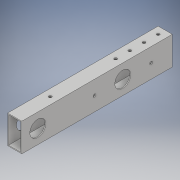
# Autodesk Inventor part: 1X2 7in
Saved by Autodesk Inventor 2018 (Build 220112000, 112)
## iProperties
Created: 2019-01-11
Material: Generic
Document SubType Name: Modeling
Designer: s-2512711
Density: 1 g/cm^3
Appearance: Default
Author: s-2512711
Autodesk Inventor part; units mm, degrees
ref_plane "YZ Plane" through (0, 0, 0) normal (1, 0, 0) x (0, 1, 0)
ref_plane "XZ Plane" through (0, 0, 0) normal (0, 1, 0) x (-1, 0, 0)
ref_plane "XY Plane" through (0, 0, 0) normal (0, 0, 1) x (1, 0, 0)
sketch "Sketch1" plane through (0, 0, 0) normal (0, 0, 1) x (1, 0, 0)
  line L0 (0, 0) -> (25.4, 0)
  line L1 (25.4, 0) -> (25.4, 50.8)
  line L2 (25.4, 50.8) -> (0, 50.8)
  line L3 (0, 50.8) -> (0, 0)
  line L4 (1.5875, 49.2125) -> (23.8125, 49.2125)
  line L5 (23.8125, 49.2125) -> (23.8125, 1.5875)
  line L6 (23.8125, 1.5875) -> (1.5875, 1.5875)
  line L7 (1.5875, 1.5875) -> (1.5875, 49.2125)
  dimension "d0" = 25.4
  dimension "d1" = 50.8
  dimension "d2" = 1.5875
  constraints: 16 end point, 4 parallel, 2 perpendicular, 1 horizontal, 3 other
  measures "d0" distance of L2.end L1.end
  measures "d1" distance of L1.end L0.end
  measures "d2" distance between parallel lines of L2 L4
extrude "Extrusion1" add sketch "Sketch1" along normal blind 269.875
sketch "Sketch2" plane through (25.4, 0, 0) normal (1, 0, 0) x (0, 0, -1)
  line L0 (-269.875, 49.2125) -> (-269.875, 1.5875) construction
  line L1 (-269.875, 25.4) -> (-241.3, 25.4) construction
  circle A0 centre (-241.3, 25.4) radius 14.2875
  point P0 (0, 0)
  dimension "d20" = 28.575
  dimension "d21" = 28.575
  constraints: 2 end point, 1 centre point, 1 coincident, 1 horizontal, 1 midpoint
  measures "d20" distance of L1.start L1.end
  measures "d21" diameter of A0
sketch "Sketch4" plane through (0, 50.8, 0) normal (0, 1, 0) x (1, 0, 0)
  line L0 (1.5875, 0) -> (23.8125, 0) construction
  line L1 (12.7, 0) -> (12.7, -12.7) construction
  line L2 (12.7, -12.7) -> (12.7, -38.1) construction
  line L3 (12.7, -38.1) -> (12.7, -63.5) construction
  circle A0 centre (12.7, -12.7) radius 2.5797
  circle A1 centre (12.7, -38.1) radius 2.5797
  circle A2 centre (12.7, -63.5) radius 2.5797
  point P0 (0, 0)
  dimension "d14" = 12.7
  dimension "d15" = 25.4
  dimension "d16" = 25.4
  dimension "d17" = 5.1594
  constraints: 6 end point, 3 centre point, 3 coincident, 2 point on line, 1 midpoint, 1 vertical
  measures "d14" distance of L1.start L1.end
  measures "d15" distance of L1.end L2.end
  measures "d16" distance of L2.end L3.end
  measures "d17" diameter of A0
extrude "Extrusion4" cut sketch "Sketch4" against normal blind 68.2625
extrude "Extrusion5" cut sketch "Sketch2" against normal blind 25.4
sketch "Sketch5" plane through (25.4, 0, 0) normal (1, 0, 0) x (0, 0, -1)
  line L0 (0, 1.5875) -> (0, 49.2125) construction
  line L1 (0, 25.4) -> (-38.1, 25.4) construction
  line L2 (0, 25.4) -> (38.1, 25.4) construction
  line L3 (-38.1, 25.4) -> (-139.7, 25.4) construction
  circle A0 centre (-139.7, 25.4) radius 2.5797
  circle A1 centre (-38.1, 25.4) radius 2.5797
  circle A2 centre (-88.9, 25.4) radius 14.2875
  point P0 (0, 0)
  dimension "d24" = 38.1
  dimension "d25" = 180
  dimension "d26" = 101.6
  dimension "d27" = 5.1594
  dimension "d30" = 28.575
  constraints: 6 end point, 3 centre point, 3 horizontal, 2 coincident, 2 midpoint, 1 collinear
  measures "d24" distance of L1.start L1.end
  measures "d25" angle of L1 L2
  measures "d26" distance of L1.end L3.end
  measures "d27" diameter of A0
  measures "d30" diameter of A2
extrude "Extrusion7" cut sketch "Sketch5" against normal blind 25.4
sketch "Sketch7" plane through (0, 50.8, 0) normal (0, 1, 0) x (1, 0, 0)
  circle A0 centre (12.7, -63.5) radius 2.5797 construction
  line L0 (12.7, -63.5) -> (12.7, -88.9) construction
  circle A1 centre (12.7, -88.9) radius 2.5797
  point P0 (0, 0)
  dimension "d37" = 25.4
  constraints: 2 end point, 1 centre point, 1 coincident, 1 vertical
  measures "d37" distance of L0.start L0.end
extrude "Extrusion9" cut sketch "Sketch7" against normal blind 66.675
sketch "Sketch8" plane through (0, 50.8, 0) normal (0, 1, 0) x (1, 0, 0)
  line L0 (23.8125, -269.875) -> (1.5875, -269.875) construction
  line L1 (12.7, -269.875) -> (12.7, -206.375) construction
  circle A0 centre (12.7, -206.375) radius 2.5797
  point P0 (0, 0)
  dimension "d40" = 63.5
  dimension "d41" = 5.1594
  constraints: 2 end point, 1 centre point, 1 coincident, 1 midpoint, 1 vertical
  measures "d40" distance of L1.start L1.end
  measures "d41" diameter of A0
extrude "Extrusion10" cut sketch "Sketch8" against normal blind 66.675
body "Solid1"
